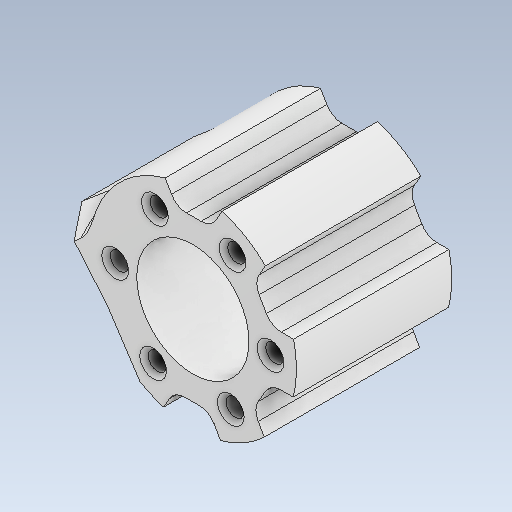
# Autodesk Inventor part: joint_connector_1
Saved by Autodesk Inventor 2020 (Build 240168000, 168)
## iProperties
Created: 2020-08-28
Part Number: joint_connector_1
Material: ABS Plastic
Document SubType Name: Modeling
Designer: psrobotics
Density: 1.06 g/cm^3
Appearance: Smooth - White
Author: psrobotics
Autodesk Inventor part; units mm, degrees
ref_plane "YZ Plane" through (0, 0, 0) normal (1, 0, 0) x (0, 1, 0)
sketch "Sketch1" plane through (0, 0, 0) normal (0, 0, 1) x (1, 0, 0)
  line L0 (41.6789, 41.5803) -> (38.3875, 41.1183) projected
  arc A0 (35.9812, 41.8436) -> (38.3875, 41.1183) centre (37.9705, 44.0892) ccw projected
  arc A1 (35.9812, 41.8436) -> (31.1056, 45.6861) centre (0.1733, 1.4234) ccw projected
  arc A2 (31.9732, 49.3061) -> (31.1056, 45.6861) centre (32.2512, 47.3255) ccw projected
  line L1 (31.9732, 49.3061) -> (42.9792, 50.8511) projected
  arc A3 (45.1659, 48.2729) -> (42.9792, 50.8511) centre (43.2572, 48.8706) ccw projected
  arc A4 (45.1659, 48.2729) -> (44.2325, 44.1325) centre (69.978, 40.504) ccw projected
  arc A5 (41.6789, 41.5803) -> (44.2325, 44.1325) centre (41.2618, 44.5512) ccw projected
  circle A6 centre (69.978, 40.504) radius 10 projected
  arc A7 (39.2456, 28.4345) -> (37.346, 30.9943) centre (0.1733, 1.4234) ccw projected
  arc A8 (38.1958, 24.0848) -> (39.2456, 28.4345) centre (36.7779, 26.7286) ccw projected
  line L2 (38.1958, 24.0848) -> (31.5355, 20.5128) projected
  arc A9 (27.6897, 21.3945) -> (31.5355, 20.5128) centre (30.1177, 23.1566) ccw projected
  arc A10 (27.6897, 21.3945) -> (27.5008, 21.6522) centre (0.1733, 1.4234) ccw projected
  arc A11 (27.6755, 25.4365) -> (27.5008, 21.6522) centre (29.9121, 23.4371) ccw projected
  line L3 (27.6755, 25.4365) -> (32.7616, 31.1261) projected
  arc A12 (37.346, 30.9943) -> (32.7616, 31.1261) centre (34.9982, 29.1267) ccw projected
  arc A13 (17.2245, 30.8386) -> (15.3151, 31.8656) centre (0.1733, 1.4234) ccw projected
  arc A14 (13.8655, 35.6655) -> (15.3151, 31.8656) centre (16.6511, 34.5516) ccw projected
  line L4 (13.8655, 35.6655) -> (16.6578, 42.6485) projected
  arc A15 (20.7425, 44.2388) -> (16.6578, 42.6485) centre (19.4434, 41.5346) ccw projected
  arc A16 (25.409, 41.6652) -> (20.7425, 44.2388) centre (0.1733, 1.4234) ccw projected
  arc A17 (26.0518, 37.1243) -> (25.409, 41.6652) centre (23.8152, 39.1236) ccw projected
  line L5 (26.0518, 37.1243) -> (20.9656, 31.4347) projected
  arc A18 (17.2245, 30.8386) -> (20.9656, 31.4347) centre (18.729, 33.4341) ccw projected
  circle A19 centre (61.1849, 56.2101) radius 2 projected
  circle A20 centre (79.1833, 55.9721) radius 2 projected
  circle A21 centre (87.9764, 40.2661) radius 2 projected
  circle A22 centre (78.7712, 24.7979) radius 2 projected
  circle A23 centre (60.7727, 25.0359) radius 2 projected
  circle A24 centre (51.9796, 40.742) radius 2 projected
  circle A25 centre (-39.2427, 1.4435) radius 2.05 projected
  circle A26 centre (-33.5273, 15.312) radius 2.05 projected
  circle A27 centre (-27.8118, 29.1804) radius 2.05 projected
  line L6 (-6.6144, -39.5468) -> (-4.9218, -40.8928) projected
  arc A28 (-5.7012, -44.4033) -> (-4.9218, -40.8928) centre (-6.1666, -42.4582) ccw projected
  line L7 (-5.7012, -44.4033) -> (-8.0919, -44.9753) projected
  arc A29 (-10.4367, -42.3462) -> (-8.0919, -44.9753) centre (-8.5573, -43.0302) ccw projected
  line L8 (-10.4367, -42.3462) -> (-9.7386, -40.4282) projected
  arc A30 (-6.6144, -39.5468) -> (-9.7386, -40.4282) centre (-7.8592, -41.1122) ccw projected
  line L9 (45.8812, 17.2926) -> (46.4911, 13.9051) projected
  arc A31 (43.208, 12.0435) -> (46.4911, 13.9051) centre (44.5227, 13.5507) ccw projected
  line L10 (43.208, 12.0435) -> (40.5709, 14.3438) projected
  arc A32 (40.9403, 17.6135) -> (40.5709, 14.3438) centre (41.8856, 15.851) ccw projected
  line L11 (40.9403, 17.6135) -> (42.9676, 18.7008) projected
  arc A33 (45.8812, 17.2926) -> (42.9676, 18.7008) centre (43.9129, 16.9383) ccw projected
  arc A34 (5.08, 48.6693) -> (-2.4, 48.8536) centre (0.1733, 1.4234) ccw projected
  arc A35 (7.7264, 45.175) -> (5.08, 48.6693) centre (4.7701, 45.6853) ccw projected
  line L12 (7.7264, 45.175) -> (6.447, 37.764) projected
  arc A36 (3.2217, 35.2865) -> (6.447, 37.764) centre (3.4907, 38.2744) ccw projected
  arc A37 (3.2217, 35.2865) -> (-0.8096, 35.4092) centre (0.1733, 1.4234) ccw projected
  arc A38 (-3.8489, 37.8764) -> (-0.8096, 35.4092) centre (-0.8963, 38.4079) ccw projected
  line L13 (-3.8489, 37.8764) -> (-5.1901, 45.3265) projected
  arc A39 (-2.4, 48.8536) -> (-5.1901, 45.3265) centre (-2.2375, 45.858) ccw projected
  line L14 (-12.4398, -33.2308) -> (-15.012, -40.2978) projected
  arc A40 (-19.0449, -42.0152) -> (-15.012, -40.2978) centre (-17.8311, -39.2717) ccw projected
  arc A41 (-31.0736, -34.3521) -> (-19.0449, -42.0152) centre (0.1733, 1.4234) ccw projected
  arc A42 (-31.2214, -29.9713) -> (-31.0736, -34.3521) centre (-29.1001, -32.0926) ccw projected
  line L15 (-31.2214, -29.9713) -> (-25.9036, -24.6534) projected
  arc A43 (-21.8399, -24.4884) -> (-25.9036, -24.6534) centre (-23.7822, -26.7747) ccw projected
  arc A44 (-21.8399, -24.4884) -> (-14.0077, -29.4781) centre (0.1733, 1.4234) ccw projected
  arc A45 (-12.4398, -33.2308) -> (-14.0077, -29.4781) centre (-15.2589, -32.2047) ccw projected
  line L16 (-30.7554, -18.6619) -> (-37.0627, -22.7579) projected
  arc A46 (-41.317, -21.7025) -> (-37.0627, -22.7579) centre (-38.6966, -20.2419) ccw projected
  arc A47 (-44.775, -13.9357) -> (-41.317, -21.7025) centre (0.1733, 1.4234) ccw projected
  arc A48 (-42.7127, -10.0678) -> (-44.775, -13.9357) centre (-41.9362, -12.9656) ccw projected
  line L17 (-42.7127, -10.0678) -> (-35.4483, -8.1214) projected
  arc A49 (-31.8466, -10.0103) -> (-35.4483, -8.1214) centre (-34.6719, -11.0192) ccw projected
  arc A50 (-31.8466, -10.0103) -> (-29.7491, -14.7214) centre (0.1733, 1.4234) ccw projected
  arc A51 (-30.7554, -18.6619) -> (-29.7491, -14.7214) centre (-32.3893, -16.1459) ccw projected
  line L18 (-10.111, 44.4407) -> (-8.7698, 36.9905) projected
  arc A52 (-10.7578, 33.6183) -> (-8.7698, 36.9905) centre (-11.7223, 36.459) ccw projected
  arc A53 (-10.7578, 33.6183) -> (-14.4933, 32.0974) centre (0.1733, 1.4234) ccw projected
  arc A54 (-18.3801, 33.2946) -> (-14.4933, 32.0974) centre (-15.7874, 34.8039) ccw projected
  line L19 (-18.3801, 33.2946) -> (-22.1637, 39.7941) projected
  arc A55 (-20.902, 43.992) -> (-22.1637, 39.7941) centre (-19.571, 41.3034) ccw projected
  arc A56 (-13.9559, 46.7733) -> (-20.902, 43.992) centre (0.1733, 1.4234) ccw projected
  arc A57 (-10.111, 44.4407) -> (-13.9559, 46.7733) centre (-13.0635, 43.9091) ccw projected
  line L20 (14.2914, 9.8007) -> (19.335, 18.2488) projected
  arc A58 (21.8027, 18.4062) -> (19.335, 18.2488) centre (20.6229, 17.4799) ccw projected
  arc A59 (26.4331, 9.5885) -> (21.8027, 18.4062) centre (0.1733, 1.4234) ccw projected
  arc A60 (24.9026, 7.6464) -> (26.4331, 9.5885) centre (25.0008, 9.1432) ccw projected
  line L21 (24.9026, 7.6464) -> (15.0846, 8.2903) projected
  arc A61 (14.2914, 9.8007) -> (15.0846, 8.2903) centre (15.1501, 9.2881) ccw projected
  line L22 (16.08, -2.636) -> (25.62, -0.2287) projected
  arc A62 (27.4763, -1.8623) -> (25.62, -0.2287) centre (25.987, -1.6831) ccw projected
  arc A63 (24.5154, -11.3715) -> (27.4763, -1.8623) centre (0.1733, 1.4234) ccw projected
  arc A64 (22.0599, -11.6626) -> (24.5154, -11.3715) centre (23.1877, -10.6736) ccw projected
  line L23 (22.0599, -11.6626) -> (15.5728, -4.2649) projected
  arc A65 (16.08, -2.636) -> (15.5728, -4.2649) centre (16.3246, -3.6056) ccw projected
  line L24 (8.5506, -12.6948) -> (16.9986, -17.7383) projected
  arc A66 (17.1561, -20.2061) -> (16.9986, -17.7383) centre (16.2297, -19.0263) ccw projected
  arc A67 (8.3384, -24.8365) -> (17.1561, -20.2061) centre (0.1733, 1.4234) ccw projected
  arc A68 (6.3962, -23.3059) -> (8.3384, -24.8365) centre (7.893, -23.4041) ccw projected
  line L25 (6.3962, -23.3059) -> (7.0401, -13.488) projected
  arc A69 (8.5506, -12.6948) -> (7.0401, -13.488) centre (8.038, -13.5534) ccw projected
  line L26 (-3.8861, -14.4833) -> (-1.4788, -24.0233) projected
  arc A70 (-3.1124, -25.8796) -> (-1.4788, -24.0233) centre (-2.9332, -24.3904) ccw projected
  arc A71 (-12.6216, -22.9188) -> (-3.1124, -25.8796) centre (0.1733, 1.4234) ccw projected
  arc A72 (-12.9127, -20.4632) -> (-12.6216, -22.9188) centre (-11.9237, -21.591) ccw projected
  line L27 (-12.9127, -20.4632) -> (-5.5151, -13.9761) projected
  arc A73 (-3.8861, -14.4833) -> (-5.5151, -13.9761) centre (-4.8558, -14.728) ccw projected
  line L28 (-13.9449, -6.9539) -> (-18.9885, -15.402) projected
  arc A74 (-21.4562, -15.5594) -> (-18.9885, -15.402) centre (-20.2764, -14.6331) ccw projected
  arc A75 (-26.0866, -6.7418) -> (-21.4562, -15.5594) centre (0.1733, 1.4234) ccw projected
  arc A76 (-24.5561, -4.7996) -> (-26.0866, -6.7418) centre (-24.6543, -6.2964) ccw projected
  line L29 (-24.5561, -4.7996) -> (-14.7381, -5.4435) projected
  arc A77 (-13.9449, -6.9539) -> (-14.7381, -5.4435) centre (-14.8035, -6.4413) ccw projected
  line L30 (-15.7335, 5.4828) -> (-25.2735, 3.0755) projected
  arc A78 (-27.1298, 4.7091) -> (-25.2735, 3.0755) centre (-25.6405, 4.5299) ccw projected
  arc A79 (-24.1689, 14.2183) -> (-27.1298, 4.7091) centre (0.1733, 1.4234) ccw projected
  arc A80 (-21.7134, 14.5094) -> (-24.1689, 14.2183) centre (-22.8412, 13.5204) ccw projected
  line L31 (-21.7134, 14.5094) -> (-15.2263, 7.1117) projected
  arc A81 (-15.7335, 5.4828) -> (-15.2263, 7.1117) centre (-15.9781, 6.4524) ccw projected
  line L32 (-8.2041, 15.5416) -> (-16.6521, 20.5851) projected
  arc A82 (-16.8096, 23.0529) -> (-16.6521, 20.5851) centre (-15.8832, 21.8731) ccw projected
  arc A83 (-7.9919, 27.6833) -> (-16.8096, 23.0529) centre (0.1733, 1.4234) ccw projected
  arc A84 (-6.0497, 26.1527) -> (-7.9919, 27.6833) centre (-7.5465, 26.2509) ccw projected
  line L33 (-6.0497, 26.1527) -> (-6.6936, 16.3348) projected
  arc A85 (-8.2041, 15.5416) -> (-6.6936, 16.3348) centre (-7.6915, 16.4002) ccw projected
  line L34 (4.2326, 17.3301) -> (1.8253, 26.8701) projected
  arc A86 (3.4589, 28.7264) -> (1.8253, 26.8701) centre (3.2797, 27.2372) ccw projected
  arc A87 (12.9681, 25.7656) -> (3.4589, 28.7264) centre (0.1733, 1.4234) ccw projected
  arc A88 (13.2592, 23.31) -> (12.9681, 25.7656) centre (12.2702, 24.4378) ccw projected
  line L35 (13.2592, 23.31) -> (5.8616, 16.8229) projected
  arc A89 (4.2326, 17.3301) -> (5.8616, 16.8229) centre (5.2023, 17.5748) ccw projected
  circle A90 centre (-10.0674, -10.8701) radius 2 projected
  circle A91 centre (10.4139, 13.7169) radius 2 projected
  circle A92 centre (15.1114, 2.7842) radius 1.5 projected
  circle A93 centre (-14.7649, 0.0626) radius 1.5 projected
  circle A94 centre (1.5341, -13.5147) radius 1.5 projected
  circle A95 centre (-1.1876, 16.3615) radius 1.5 projected
  circle A96 centre (12.4667, -8.8173) radius 2 projected
  circle A97 centre (-12.1202, 11.664) radius 2 projected
  circle A98 centre (0.1733, 1.4234) radius 12 projected
  circle A99 centre (18.3916, 52.0411) radius 1.55 projected
  circle A100 centre (-53.4988, -8.0404) radius 1.55 projected
  circle A101 centre (-29.775, -44.1107) radius 1.55 projected
  circle A102 centre (-9.2906, -52.2486) radius 1.55 projected
  circle A103 centre (-45.3608, -28.5248) radius 1.55 projected
  circle A104 centre (-34.5538, 42.5098) radius 1.55 projected
  circle A105 centre (53.1186, 10.9547) radius 1.55 projected
  line L36 (5.4722, -42.7701) -> (-1.7065, -37.0615) projected
  arc A106 (0.4203, -29.9472) -> (-1.7065, -37.0615) centre (0.7832, -33.9307) ccw projected
  line L37 (0.4203, -29.9472) -> (18.0587, -28.3404) projected
  line L38 (32.7441, -11.5046) -> (18.0587, -28.3404) projected
  line L39 (32.7441, -11.5046) -> (31.0721, 6.849) projected
  arc A107 (37.685, 10.2263) -> (31.0721, 6.849) centre (35.0556, 7.2119) ccw projected
  line L40 (37.685, 10.2263) -> (45.6437, 3.2841) projected
  line L41 (47.8942, 5.8641) -> (45.6437, 3.2841) projected
  arc A108 (49.1938, 6.5386) -> (47.8942, 5.8641) centre (49.4014, 4.5494) ccw projected
  line L42 (53.8816, 7.0278) -> (49.1938, 6.5386) projected
  line L43 (57.764, 7.7267) -> (53.8816, 7.0278) projected
  line L44 (57.764, 7.7267) -> (80.5887, 18.977) projected
  arc A109 (80.5887, 18.977) -> (66.6416, 64.271) centre (69.978, 40.504) ccw projected
  line L45 (66.6416, 64.271) -> (15.9826, 57.1593) projected
  line L46 (15.5667, 56.004) -> (15.9826, 57.1593) projected
  arc A110 (12.0824, 54.0938) -> (15.5667, 56.004) centre (12.744, 57.0199) ccw projected
  arc A111 (12.0824, 54.0938) -> (0.5596, 55.422) centre (0.1733, 1.4234) ccw projected
  arc A112 (-1.2772, 56.0668) -> (0.5596, 55.422) centre (0.5811, 58.4219) ccw projected
  line L47 (-17.5237, 53.1421) -> (-1.2772, 56.0668) projected
  arc A113 (-19.0204, 51.8972) -> (-17.5237, 53.1421) centre (-20.0867, 54.7013) ccw projected
  arc A114 (-19.0204, 51.8972) -> (-29.3565, 46.6339) centre (0.1733, 1.4234) ccw projected
  arc A115 (-33.2883, 47.209) -> (-29.3565, 46.6339) centre (-30.9971, 49.1456) ccw projected
  line L48 (-34.0809, 48.1469) -> (-33.2883, 47.209) projected
  line L49 (-40.1908, 42.9826) -> (-34.0809, 48.1469) projected
  line L50 (-37.6444, 39.9698) -> (-40.1908, 42.9826) projected
  line L51 (-34.7161, 36.9851) -> (-37.6444, 39.9698) projected
  arc A116 (-34.2938, 34.8242) -> (-34.7161, 36.9851) centre (-36.1437, 35.5844) ccw projected
  line L52 (-49.2479, -1.5605) -> (-34.2938, 34.8242) projected
  arc A117 (-50.7504, -2.7699) -> (-49.2479, -1.5605) centre (-51.0977, -0.8002) ccw projected
  line L53 (-57.764, -4.0066) -> (-50.7504, -2.7699) projected
  line L54 (-56.251, -12.5874) -> (-57.764, -4.0066) projected
  line L55 (-53.9639, -12.1842) -> (-56.251, -12.5874) projected
  arc A118 (-51.6956, -13.5974) -> (-53.9639, -12.1842) centre (-53.6166, -14.1538) ccw projected
  arc A119 (-51.6956, -13.5974) -> (-47.8627, -23.2454) centre (0.1733, 1.4234) ccw projected
  arc A120 (-48.5428, -25.83) -> (-47.8627, -23.2454) centre (-49.6418, -24.159) ccw projected
  line L56 (-50.4831, -27.1062) -> (-48.5428, -25.83) projected
  line L57 (-46.087, -33.7901) -> (-50.4831, -27.1062) projected
  line L58 (-44.1467, -32.5139) -> (-46.087, -33.7901) projected
  arc A121 (-41.5041, -32.9132) -> (-44.1467, -32.5139) centre (-43.0477, -34.1849) ccw projected
  arc A122 (-41.5041, -32.9132) -> (-34.1633, -40.2539) centre (0.1733, 1.4234) ccw projected
  arc A123 (-33.7641, -42.8966) -> (-34.1633, -40.2539) centre (-35.435, -41.7975) ccw projected
  line L59 (-35.0402, -44.8369) -> (-33.7641, -42.8966) projected
  line L60 (-28.3563, -49.2329) -> (-35.0402, -44.8369) projected
  line L61 (-27.0802, -47.2926) -> (-28.3563, -49.2329) projected
  arc A124 (-24.4955, -46.6125) -> (-27.0802, -47.2926) centre (-25.4092, -48.3917) ccw projected
  arc A125 (-24.4955, -46.6125) -> (-14.8476, -50.4454) centre (0.1733, 1.4234) ccw projected
  arc A126 (-13.4343, -52.7138) -> (-14.8476, -50.4454) centre (-15.4039, -52.3665) ccw projected
  line L62 (-13.8376, -55.0009) -> (-13.4343, -52.7138) projected
  line L63 (-1.5962, -57.1593) -> (-13.8376, -55.0009) projected
  line L64 (-0.3036, -49.8289) -> (-1.5962, -57.1593) projected
  arc A127 (0.1588, -48.8615) -> (-0.3036, -49.8289) centre (1.666, -50.1762) ccw projected
  line L65 (5.4722, -42.7701) -> (0.1588, -48.8615) projected
  circle A128 centre (69.978, 40.504) radius 13
  circle A129 centre (69.978, 40.504) radius 24
  point P0 (0, 0)
  point P1 (66.6416, 64.271)
  dimension "d0" = 26
  dimension "d1" = 48
  constraints: 2 centre point, 2 coincident
  measures "d0" diameter of A128
  measures "d1" diameter of A129
ref_plane "Work Plane1" through (-7.4404, -12.529, 36) normal (0, 0, -1) x (0.6400405, 0.7683411, 0)
extrude "Extrusion1" add sketch "Sketch1" along normal up to surface (36 mm away) contours A129 A109
sketch "Sketch2" plane through (69.978, 40.504, 36) normal (0, 0, 1) x (1, 0, 0)
  circle A0 centre (0, 0) radius 13 projected
  circle A1 centre (-17.9984, 0.238) radius 2 projected
  circle A2 centre (-9.2053, -15.4681) radius 2 projected
  circle A3 centre (8.7931, -15.7061) radius 2 projected
  circle A4 centre (17.9984, -0.238) radius 2 projected
  circle A5 centre (9.2053, 15.4681) radius 2 projected
  circle A6 centre (-8.7931, 15.7061) radius 2 projected
  circle A7 centre (0, 0) radius 24 projected
  point P0 (-69.978, -40.504)
hole "Hole1" at (61.1849, 56.2101, 36) at (79.1833, 55.9721, 36) at (87.9764, 40.2661, 36) at (78.7712, 24.7979, 36) at (60.7727, 25.0359, 36) at (51.9796, 40.742, 36) direction (0, 0, -1) diameter 4.2 end through all
chamfer "Chamfer1" distance 1 angle 45 12 edges at (61.1849, 58.3101, 36) (79.1833, 58.0721, 36) (87.9764, 42.3661, 36) (78.7712, 26.8979, 36) (60.7727, 27.1359, 36) (51.9796, 42.842, 36) (87.9764, 42.3661, 0) (79.1833, 58.0721, 0) (61.1849, 58.3101, 0) (51.9796, 42.842, 0) (60.7727, 27.1359, 0) (78.7712, 26.8979, 0)
sketch "Sketch3" plane through (69.978, 40.504, 36) normal (0, 0, 1) x (1, 0, 0)
  circle A0 centre (-16.8594, -29.5493) radius 2.05 projected
  circle A1 centre (-51.5864, 11.5371) radius 2.05 projected
  circle A2 centre (-104.5318, 2.0058) radius 2.05 projected
  line L0 (-107.6224, -0.5342) -> (-103.7706, -4.4602) projected
  arc A3 (-21.5667, -34.0471) -> (-103.7706, -4.4602) centre (-69.8048, -39.0806) ccw projected
  line L1 (-21.5667, -34.0471) -> (-16.0964, -33.4763) projected
  line L2 (-12.214, -32.7773) -> (-16.0964, -33.4763) projected
  line L3 (-13.6314, -24.9039) -> (-12.214, -32.7773) projected
  line L4 (-14.8399, -25.1215) -> (-13.6314, -24.9039) projected
  arc A4 (-18.2363, -23.059) -> (-14.8399, -25.1215) centre (-15.3714, -22.1689) ccw projected
  arc A5 (-18.2363, -23.059) -> (-22.8474, -12.4159) centre (-69.8048, -39.0806) ccw projected
  arc A6 (-22.1752, -8.6433) -> (-22.8474, -12.4159) centre (-20.2387, -10.9345) ccw projected
  line L5 (-22.1752, -8.6433) -> (-21.0484, -7.6909) projected
  line L6 (-21.0484, -7.6909) -> (-30.7313, 3.7652) projected
  line L7 (-30.7313, 3.7652) -> (-31.8581, 2.8127) projected
  arc A7 (-35.69, 2.7785) -> (-31.8581, 2.8127) centre (-33.7947, 5.104) ccw projected
  arc A8 (-35.69, 2.7785) -> (-45.4162, 9.0982) centre (-69.8048, -39.0806) ccw projected
  arc A9 (-46.884, 12.7908) -> (-45.4162, 9.0982) centre (-44.0613, 11.7748) ccw projected
  line L8 (-46.4682, 13.9461) -> (-46.884, 12.7908) projected
  line L9 (-53.9955, 16.6553) -> (-46.4682, 13.9461) projected
  line L10 (-54.4113, 15.5) -> (-53.9955, 16.6553) projected
  arc A10 (-57.8956, 13.5898) -> (-54.4113, 15.5) centre (-57.234, 16.5159) ccw projected
  arc A11 (-57.8956, 13.5898) -> (-69.4184, 14.918) centre (-69.8048, -39.0806) ccw projected
  arc A12 (-72.3495, 17.3864) -> (-69.4184, 14.918) centre (-69.3969, 17.9179) ccw projected
  line L11 (-72.3495, 17.3864) -> (-72.6109, 18.8385) projected
  line L12 (-72.6109, 18.8385) -> (-87.3736, 16.1809) projected
  line L13 (-87.3736, 16.1809) -> (-87.1122, 14.7288) projected
  arc A13 (-88.9984, 11.3932) -> (-87.1122, 14.7288) centre (-90.0647, 14.1973) ccw projected
  arc A14 (-88.9984, 11.3932) -> (-99.3345, 6.1299) centre (-69.8048, -39.0806) ccw projected
  arc A15 (-103.2663, 6.705) -> (-99.3345, 6.1299) centre (-100.9751, 8.6416) ccw projected
  line L14 (-104.059, 7.6428) -> (-103.2663, 6.705) projected
  line L15 (-110.1689, 2.4786) -> (-104.059, 7.6428) projected
  line L16 (-107.6224, -0.5342) -> (-110.1689, 2.4786) projected
  circle A16 centre (-9.2053, -15.4681) radius 3.1 projected
  circle A17 centre (17.9984, -0.238) radius 3.1 projected
  circle A18 centre (-8.7931, 15.7061) radius 3.1 projected
  circle A19 centre (0, 0) radius 13 projected
  circle A20 centre (0, 0) radius 24 projected
  circle A21 centre (9.2053, 15.4681) radius 3.1 projected
  circle A22 centre (8.7931, -15.7061) radius 3.1 projected
  circle A23 centre (-17.9984, 0.238) radius 3.1 projected
  line L17 (-21.0484, -7.6909) -> (-19.7573, -9.2184)
  line L18 (-19.7573, -9.2184) -> (-22.1752, -11.262)
  line L19 (-22.1752, -11.262) -> (-22.8474, -12.4159)
  point P0 (-69.978, -40.504)
  point P1 (-23.5225, -4.7637)
  point P2 (-21.4909, -10.6836)
  dimension "d14" = 2
  constraints: 6 end point, 1 collinear, 1 perpendicular
  measures "d14" distance of L5.end L17.end
extrude "Extrusion2" cut sketch "Sketch3" against normal blind 50 contours A20 L6 L5 A6 | A6 L5 L17 L18 A20
sketch "Sketch4" plane through (69.978, 40.504, 36) normal (0, 0, 1) x (0.9458545, 0.324591, 0)
  line L0 (-21.6798, -2.3062) -> (-23.7951, -3.1294) projected
  arc A0 (-23.7951, -3.1294) -> (-23.7951, 3.1294) centre (0, 0) ccw projected
  line L1 (-23.7951, 3.1294) -> (-21.6798, -2.3062) projected
  circle A1 centre (-13.7277, -11.6426) radius 3.1 projected
  circle A2 centre (16.9467, -6.0672) radius 3.1 projected
  circle A3 centre (-3.219, 17.7098) radius 3.1 projected
  circle A4 centre (0, 0) radius 13 projected
  circle A5 centre (13.7277, 11.6426) radius 3.1 projected
  circle A6 centre (3.219, -17.7098) radius 3.1 projected
  circle A7 centre (-16.9467, 6.0672) radius 3.1 projected
  line L2 (-25.6691, 7.9449) -> (-27.8452, 13.5364) projected
  line L3 (-24.5811, 5.1492) -> (-25.6691, 7.9449) projected
  line L4 (-22.4051, -0.4423) -> (-24.5811, 5.1492) projected
  line L5 (-27.8452, 13.5364) -> (-15.462, 18.3555)
  arc A8 (-23.7951, -3.1294) -> (-23.7951, 3.1294) centre (0, 0) ccw projected
  point P0 (-79.3363, -15.5967)
  point P1 (-15.462, 18.3555)
  constraints: 2 end point, 1 perpendicular, 1 point on circle
ref_plane "Work Plane2" through (-117.5944, -131.7815, 0) normal (0, 0, 1) x (1, 0, 0)
extrude "Extrusion3" add sketch "Sketch4" against normal up to surface (36 mm away) contours A0 L4 L3 L2 L5
chamfer "Chamfer2" distance 5 angle 45 2 edges at (44.3209, 48.558, 36) (44.3209, 48.558, 0)
sketch "Sketch5" plane through (50.2207, 31.2857, 0) normal (-0.7637379, -0.6455264, 0) x (0, 0, 1)
  line L0 (2, 17) -> (2, 2) projected
  line L1 (2, 17) -> (30, 17) projected
  line L2 (30, 2) -> (30, 17) projected
  line L3 (2, 2) -> (30, 2) projected
  circle A0 centre (23, 9.5) radius 2.05 projected
  circle A1 centre (7, 9.5) radius 2.05 projected
  line L4 (17, 6.5) -> (17, 12.5) projected
  arc A2 (17, 12.5) -> (13, 12.5) centre (15, 12.5) ccw projected
  line L5 (13, 12.5) -> (13, 6.5) projected
  arc A3 (13, 6.5) -> (17, 6.5) centre (15, 6.5) ccw projected
  circle A4 centre (23, 9.5) radius 2
  circle A5 centre (7, 9.5) radius 2
  point P0 (0, 8.5247)
  dimension "d22" = 4
  dimension "d23" = 4
  constraints: 2 centre point, 2 coincident
  measures "d22" diameter of A4
  measures "d23" diameter of A5
extrude "Extrusion4" cut sketch "Sketch5" against normal blind 10 contours A4 | A5
sketch "Sketch6" plane through (0, 0, 0) normal (0, 0, -1) x (-1, 0, 0)
  arc A0 (-46.1758, 43.5791) -> (-48.4871, 29.8204) centre (-69.978, 40.504) ccw projected
  line L0 (-48.4871, 29.8204) -> (-50.2207, 31.2857) projected
  line L1 (-50.2207, 31.2857) -> (-42.4744, 40.4505) projected
  line L2 (-46.1758, 43.5791) -> (-42.4744, 40.4505) projected
  circle A1 centre (-78.7712, 24.7979) radius 3.1 projected
  circle A2 centre (-51.9796, 40.742) radius 3.1 projected
  circle A3 centre (-79.1833, 55.9721) radius 3.1 projected
  circle A4 centre (-69.978, 40.504) radius 13 projected
  circle A5 centre (-87.9764, 40.2661) radius 3.1 projected
  circle A6 centre (-61.1849, 56.2101) radius 3.1 projected
  circle A7 centre (-60.7727, 25.0359) radius 3.1 projected
  circle A8 centre (-60.7727, 25.0359) radius 2.1 projected
  line L3 (-69.978, 40.504) -> (-60.7727, 25.0359)
  line L4 (-60.7727, 25.0359) -> (-57.7043, 19.8799)
  line L5 (-50.2207, 31.2857) -> (-57.7043, 19.8799)
  point P0 (0, 0)
  constraints: 6 end point, 1 collinear, 1 point on circle
extrude "Extrusion5" cut sketch "Sketch6" against normal blind 50 contours L5 L0 A0
sketch "Sketch7" plane through (0, 0, 0) normal (0, 0, -1) x (-1, 0, 0)
  circle A0 centre (-60.7727, 25.0359) radius 3.1 projected
  circle A1 centre (-61.1849, 56.2101) radius 3.1 projected
  circle A2 centre (-87.9764, 40.2661) radius 3.1 projected
  circle A3 centre (-69.978, 40.504) radius 13 projected
  circle A4 centre (-79.1833, 55.9721) radius 3.1 projected
  circle A5 centre (-51.9796, 40.742) radius 3.1 projected
  circle A6 centre (-78.7712, 24.7979) radius 3.1 projected
  line L0 (-57.7043, 19.8799) -> (-50.2207, 31.2857) projected
  line L1 (-50.2207, 31.2857) -> (-42.4744, 40.4505) projected
  line L2 (-46.1758, 43.5791) -> (-42.4744, 40.4505) projected
  arc A7 (-46.1758, 43.5791) -> (-57.7043, 19.8799) centre (-69.978, 40.504) ccw projected
  line L3 (-60.7727, 25.0359) -> (-78.7712, 24.7979)
  line L4 (-69.978, 40.504) -> (-69.7719, 24.9169)
  line L5 (-69.7719, 24.9169) -> (-69.7719, 21.9169)
  line L6 (-69.7719, 21.9169) -> (-73.7719, 21.9169)
  line L7 (-69.7719, 21.9169) -> (-65.7719, 21.9169)
  line L8 (-65.7719, 21.9169) -> (-63.2093, 17.4783)
  line L9 (-73.7719, 21.9169) -> (-76.3929, 17.3772)
  point P0 (0, 0)
  dimension "d28" = 3
  dimension "d29" = 4
  dimension "d30" = 4
  dimension "d31" = 120
  dimension "d32" = 120
  constraints: 14 end point, 2 horizontal, 2 point on circle, 1 midpoint, 1 vertical
  measures "d28" distance of L4.end L5.end
  measures "d29" distance of L5.end L6.end
  measures "d30" distance of L5.end L7.end
  measures "d31" angle of L6 L9
  measures "d32" angle of L7 L8
extrude "Extrusion6" cut sketch "Sketch7" against normal blind 50 contours A7 L9 L6 L7 L8
pattern_circular "Circular Pattern1" count 4 over 180 about axis through (69.978, 40.504, 0) along (0, 0, 1) of "Extrusion6"
fillet "Fillet1" radius 4 8 edges at (65.7719, 21.9169, 18) (73.7719, 21.9169, 18) (83.9719, 27.5679, 18) (87.9719, 34.4961, 18) (88.178, 46.155, 18) (84.178, 53.0832, 18) (74.1841, 59.0911, 18) (66.1841, 59.0911, 18)
fillet "Fillet2" radius 4 3 edges at (47.3069, 48.3792, 2.9359) (47.3069, 48.3792, 33.0641) (49.3951, 52.8468, 18)
chamfer "Chamfer3" distance 1 angle 45 2 edges at (44.0882, 38.5412, 5) (44.0882, 38.5412, 21)
body "Solid1"
